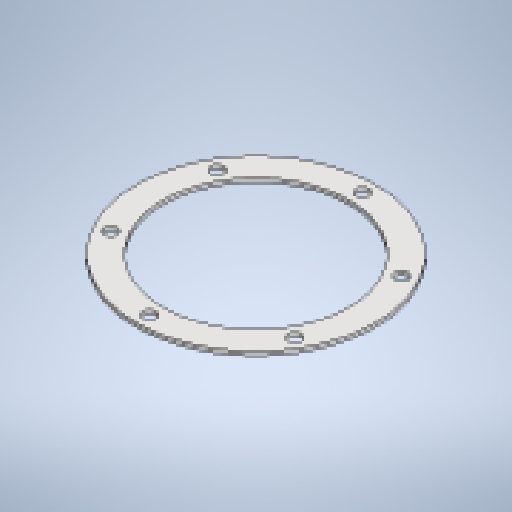
# Autodesk Inventor part: ДМФ 041 кольцо под шпильки КОРМА
Saved by Autodesk Inventor 2025 (Build 290162010, 162A)
## iProperties
Created: 2024-04-23
Part Number: ДМФ 041 кольцо под шпильки КОРМА
Material: Generic
Document SubType Name: Sheet Metal
Designer: admin
Density: 1 g/cm^3
Appearance: Default
Sheet Metal Rule: Default
Flat Pattern Width: 18 cm
Flat Pattern Length: 18 cm
Flat Pattern Area: 324 cm^2
Sheet Metal Width: 180,000 mm
Sheet Metal Length: 180,000 mm
Sheet Metal Area: 32400,000 mm^2
Stock Number: ДМФ 041 кольцо под шпильки КОРМА
back_steel_circle_диам_центров: 160,000 mm
back_steel_circle_ширина_кольца: 40,000 mm
back_steel_circle_диам_шпильки: 10,000 mm
back_steel_circle_кол_шпилек: 6,000 ul
back_steel_circle_внутр_диам: 140,000 mm
back_steel_circle_проходной_диаметр: 100,000 mm
Author: admin
Autodesk Inventor part; units mm, degrees
ref_plane "YZ Plane" through (0, 0, 0) normal (1, 0, 0) x (0, 1, 0)
ref_plane "XZ Plane" through (0, 0, 0) normal (0, 1, 0) x (-1, 0, 0)
ref_plane "XY Plane" through (0, 0, 0) normal (0, 0, 1) x (1, 0, 0)
sketch "Sketch1" plane through (0, 0, 0) normal (0, 0, 1) x (1, 0, 0)
  circle A0 centre (0, 0) radius 70
  circle A1 centre (0, 0) radius 90
  circle A2 centre (0, 0) radius 80 construction
  line L0 (0, 90) -> (0, 70) construction
  point P0 (0, 80)
  dimension "d30" = 140
  dimension "d32" = 180
extrude "Plate1" add sketch "Sketch1" along normal blind 3
sketch "Sketch2" plane through (0, 0, 3) normal (0, 0, 1) x (1, 0, 0)
  circle A0 centre (0, 0) radius 70 construction
  circle A1 centre (0, 0) radius 90 construction
  circle A2 centre (0, 0) radius 90 construction
  circle A3 centre (0, 0) radius 70 construction
  circle A4 centre (0, -80) radius 5
  circle A5 centre (0, 0) radius 80 construction
  dimension "d31" = 160
  dimension "d21" = 10
  constraints: 1 centre point, 1 coincident, 1 vertical alignment, 2 other
  measures "d21" diameter of A4
extrude "Extrusion1" cut sketch "Sketch2" against normal through all
pattern_circular "Circular Pattern2" count 6 over 360 about axis through (0, 0, 0) along (0, 0, 1) of "Extrusion1"
equation "\"d30\" = back_steel_circle_внутр_диам"
equation "\"d32\" = back_steel_circle_внутр_диам + back_steel_circle_ширина_кольца"
equation "\"d31\" = back_steel_circle_диам_центров"
equation "\"d21\" = back_steel_circle_диам_шпильки"
equation "\"d2\" = Thickness"
equation "\"BendRadius\" = Thickness"
equation "\"BendReliefWidth\" = Thickness"
equation "\"BendReliefDepth\" = 0.5 * Thickness"
equation "\"CornerReliefSize\" = 4 * Thickness"
equation "\"MinimumRemnant\" = 2 * Thickness"
equation "\"TransitionRadius\" = BendRadius"
equation "\"JacobiRadiusSize\" = BendRadius"
equation "\"GapSize\" = Thickness"
equation "\"back_steel_circle_диам_шпильки\" = 10"
equation "\"back_steel_circle_внутр_диам\" = 140"
equation "\"back_steel_circle_ширина_кольца\" = 40"
equation "\"back_steel_circle_диам_центров\" = 160"
equation "\"Thickness\" = 3"
body "Solid1"
